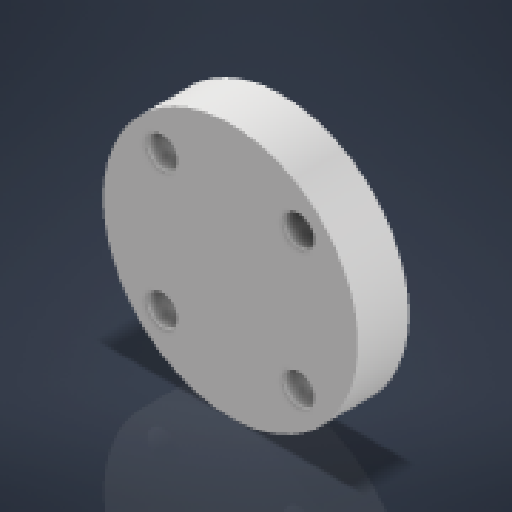
# Autodesk Inventor part: ПроставкаДвиг
Saved by Autodesk Inventor 2026 (Build 300175000, 175)
## iProperties
Created: 2025-08-20
Part Number: ПроставкаДвиг
Material: Типовые
Document SubType Name: Modeling
Designer: seraf
Density: 1 g/cm^3
Appearance: По умолчанию
Author: seraf
Autodesk Inventor part; units mm, degrees
ref_plane "YZ Plane" through (0, 0, 0) normal (1, 0, 0) x (0, 1, 0)
ref_plane "XZ Plane" through (0, 0, 0) normal (0, 1, 0) x (-1, 0, 0)
ref_plane "XY Plane" through (0, 0, 0) normal (0, 0, 1) x (1, 0, 0)
sketch "Эскиз1" plane through (0, 0, 0) normal (0, 0, 1) x (1, 0, 0)
  circle A0 centre (38.2581, 176.9621) radius 1.5 projected
  circle A1 centre (38.2581, 190.3971) radius 1.5 projected
  circle A2 centre (51.6931, 176.9621) radius 1.5 projected
  circle A3 centre (51.6931, 190.3971) radius 1.5 projected
  circle A4 centre (44.9756, 183.6796) radius 12.5 projected
  point P0 (0, 0)
extrude "Выдавливание1" add sketch "Эскиз1" along normal blind 5
